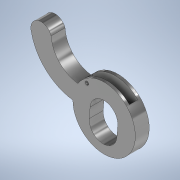
# Autodesk Inventor part: Peça_11
Saved by Autodesk Inventor 2021 (Build 250183000, 183)
## iProperties
Created: 2020-11-06
Part Number: Peça_11
Material: Liga de Nickel-Copper 400
Document SubType Name: Modeling
Designer: Bruno
Density: 8.83 g/cm^3
Appearance: Cromado - Preto polido
Author: Bruno
Autodesk Inventor part; units mm, degrees
ref_plane "YZ Plane" through (0, 0, 0) normal (1, 0, 0) x (0, 1, 0)
ref_plane "XY Plane" through (0, 0, 0) normal (0, 0, 1) x (1, 0, 0)
sketch "Esboço1" plane through (0, 0, 0) normal (0, 0, 1) x (1, 0, 0)
  circle A0 centre (0, 0) radius 4.5
  dimension "d0" = 9
  constraints: 1 centre point, 1 coincident
  measures "d0" diameter of A0
extrude "Extrusão1" add sketch "Esboço1" along normal blind 2
sketch "Esboço2" plane through (0, 0, 2) normal (0, 0, 1) x (1, 0, 0)
  circle A0 centre (0, 0) radius 4.5 projected
  arc A1 (-10.4751, 5.4783) -> (-4.5, 0.0043) centre (-3.6315, 6.9502) ccw
  arc A2 (-7.6364, 6.4456) -> (-10.4751, 5.4783) centre (-9.0687, 6) ccw
  arc A3 (-7.6364, 6.4456) -> (-3.7747, 2.4498) centre (-3.3457, 6.7283) ccw
  dimension "d3" = 7
  dimension "d4" = 4.3
  dimension "d5" = 1.5
  dimension "d6" = 6
  constraints: 8 point on circle, 3 centre point
  measures "d3" radius of A1
  measures "d4" radius of A3
  measures "d5" radius of A2
  measures "d6" vertical distance of point (0, 0) A2.centre
extrude "Extrusão2" add sketch "Esboço2" against normal blind 2 contours A0 A1 A2 A3
sketch "Esboço4" plane through (0, 0, 2) normal (0, 0, 1) x (1, 0, 0)
  line L0 (-0.335, -0.9422) -> (0.1675, 0.4711) construction
  line L1 (-2.0175, 0.3756) -> (-2.1372, -1.1196)
  line L2 (1.85, -1.439) -> (1.9698, 0.0562)
  arc A0 (1.9698, 0.0562) -> (-2.0175, 0.3756) centre (-0.0239, 0.2159) ccw
  arc A1 (-2.1372, -1.1196) -> (1.85, -1.439) centre (-0.1436, -1.2793) ccw
  point P0 (-0.0837, -0.2356)
  dimension "d11" = 1.5
  dimension "d12" = 4
  constraints: 6 end point, 4 point on circle, 4 tangent, 2 centre point, 1 midpoint, 1 parallel
  measures "d11" distance of L0.start L0.end
  measures "d12" distance between parallel lines of L2 L1
extrude "Extrusão3" cut sketch "Esboço4" against normal blind 2
ref_plane "Plano de trabalho1" through (0, 4.5, 0) normal (0, 1, 0) x (-1, 0, 0)
sketch "Esboço5" plane through (0, 4.5, 0) normal (0, 1, 0) x (-1, 0, 0)
  line L0 (-3.25, 1.6) -> (3.2747, 1.6)
  line L1 (3.2747, 1.6) -> (3.2747, 0.4)
  line L2 (3.2747, 0.4) -> (-3.25, 0.4)
  line L3 (-3.25, 0.4) -> (-3.25, 1.6)
  line L4 (-3.25, 1.6) -> (3.2747, 0.4) construction
  line L5 (3.2747, 1.6) -> (-3.25, 0.4) construction
  line L6 (4.5, 0) -> (-4.5, 0) projected
  line L7 (4.5, 2) -> (-4.5, 2) projected
  line L8 (3.7747, 0) -> (3.7747, 2) projected
  line L9 (-4.5, 2) -> (-4.5, 0)
  line L10 (-4.5, 0) -> (-4.5, 2) projected
  point P0 (0, 0)
  point P1 (0.0124, 1)
  dimension "d16" = 0.4
  dimension "d17" = 0.4
  dimension "d18" = 0.5
  dimension "d19" = 1.25
  constraints: 14 end point, 3 equal length, 2 midpoint, 1 horizontal, 1 perpendicular
  measures "d16" distance between parallel lines of L6 L2
  measures "d17" distance between parallel lines of L7 L0
  measures "d18" distance between parallel lines of L8 L1
  measures "d19" distance between parallel lines of L9 L3
extrude "Extrusão4" cut sketch "Esboço5" against normal blind 2.2 contours L0 L1 L2 L3
sketch "Esboço6" plane through (0, 0, 2) normal (0, 0, 1) x (1, 0, 0)
  circle A0 centre (-2.473, 3.141) radius 0.25
  line L0 (0, -6.9) -> (0, 9.9) projected
  line L1 (-13.5824, 0) -> (7.5137, 0) projected
  point P0 (0, 0)
  dimension "d22" = 0.5
  dimension "d28" = 2.473
  dimension "d29" = 3.141
  constraints: 1 centre point
  measures "d22" diameter of A0
  measures "d28" distance from line of L0 A0.centre
  measures "d29" distance from line of L1 A0.centre
extrude "Extrusão5" cut sketch "Esboço6" against normal blind 0.5
sketch "Esboço8" plane through (0, 2.3, 0) normal (0, 1, 0) x (1, 0, 0)
  line L0 (1.9698, -2) -> (1.9698, 0) projected
  circle A0 centre (1.9698, -1) radius 0.25
  point P0 (0, 0)
  dimension "d30" = 0.5
  constraints: 1 centre point, 1 midpoint
  measures "d30" diameter of A0
extrude "Extrusão7" cut sketch "Esboço8" against normal blind 0.1
